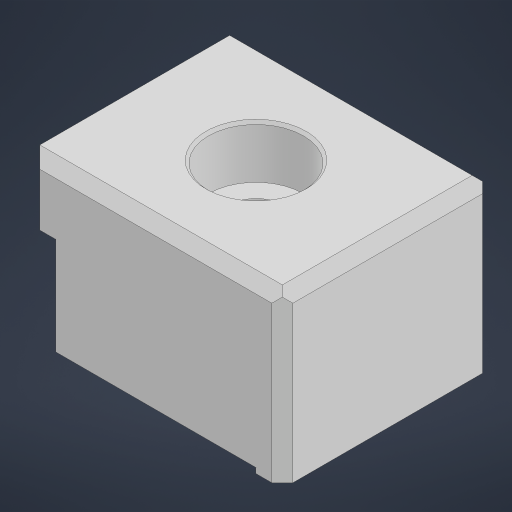
# Autodesk Inventor part: VTC1-001
Saved by Autodesk Inventor 2024.3 (Build 283343000, 343)
## iProperties
Created: 2024-02-28
Part Number: VTC1-001
Material: Generic
Document SubType Name: Modeling
Designer: fablabadmin
Density: 1 g/cm^3
Appearance: Default
Description: Clamp
Stock Number: SS1672
Author: Benjamin Solar
Revision Number: 2
Autodesk Inventor part; units mm, degrees
ref_plane "YZ Plane" through (0, 0, 0) normal (1, 0, 0) x (0, 1, 0)
ref_plane "XZ Plane" through (0, 0, 0) normal (0, 1, 0) x (-1, 0, 0)
ref_plane "XY Plane" through (0, 0, 0) normal (0, 0, 1) x (1, 0, 0)
sketch "Sketch1" plane through (0, 0, 0) normal (0, 0, 1) x (1, 0, 0)
  line L0 (-25, 15.75) -> (25, 15.75)
  line L1 (25, 15.75) -> (25, -15.75)
  line L2 (25, -15.75) -> (20, -15.75)
  line L3 (20, -15.75) -> (20, -14.75)
  line L4 (20, -14.75) -> (-18, -14.75)
  line L5 (-18, -14.75) -> (-18, 3.75)
  line L6 (-18, 3.75) -> (-25, 3.75)
  line L7 (-25, 3.75) -> (-25, 15.75)
  line L8 (-35, 0) -> (35, 0) construction
  line L9 (0, -22.05) -> (0, 22.05) construction
  point P0 (0, 0)
  dimension "d0" = 50
  dimension "d1" = 31.5
  dimension "d2" = 1
  dimension "d3" = 7
  dimension "d5" = 5
  dimension "d24" = 12
  dimension "d25" = 19.5
  constraints: 16 end point, 7 perpendicular, 1 horizontal, 2 other
  measures "d0" distance of L0.start L0.end
  measures "d1" distance of L0.end L1.end
  measures "d2" distance of L2.end L3.end
  measures "d3" distance of L5.end L6.end
  measures "d5" distance of L1.end L2.end
  measures "d24" distance of L6.end L0.start
  measures "d25" distance from line of L1.end L6
extrude "Extrusion1" add sketch "Sketch1" along normal mid plane 40
sketch "Sketch2" plane through (-25, 15.75, 20) normal (0, 1, 0) x (1, 0, 0)
  line L0 (45, 40) -> (45, 0) construction
  line L1 (7, 0) -> (45, 0) construction
  line L2 (7, 40) -> (7, 0) construction
  line L3 (45, 40) -> (7, 40) construction
  line L4 (0, 40) -> (50, 40) projected
  line L5 (25, 40) -> (25, 0)
  line L6 (50, 0) -> (0, 0) projected
  point P0 (25, 20)
  point P1 (25, 20)
  dimension "d23" = 18
  dimension "d26" = 38
  constraints: 3 midpoint, 2 end point, 1 coincident, 1 perpendicular
  measures "d23" distance between parallel lines of L2 L5
  measures "d26" distance between parallel lines of L0 L2
hole "Hole1" at (0, 15.75, 0) direction (0, -1, 0) diameter 10.5 end through all counterbore diameter 18 counterbore depth 10
chamfer "Chamfer1" distance 2 angle 45 6 edges at (-25, 15.75, 0) (0, 15.75, 20) (0, 15.75, -20) (25, 15.75, 0) (25, 0, 20) (25, 0, -20)
chamfer "Chamfer2" distance 4 angle 45 2 edges at (-25, 8.75, 20) (-25, 8.75, -20)
chamfer "Chamfer3" distance 0.5 angle 45 1 edges at (0, -14.75, -5.25)
chamfer "Chamfer4" distance 0.5 angle 45 1 edges at (0, 15.75, -9)
body "Solid1"
